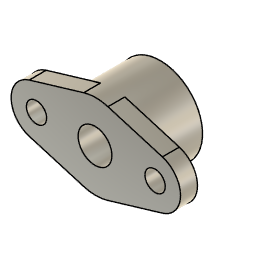
ex 4.1 v0 (Autodesk Fusion 360 design; units mm, degrees)
Autodesk Fusion 360 part; units mm, degrees
sketch "Sketch1" plane through (0, 0, 0) normal (0, 1, 0) x (1, 0, 0)
  circle A0 centre (0, 0) radius 25
  line L0 (20, 0) -> (35, 0)
  line L1 (7.1429, -23.9579) -> (39.2857, -14.3747)
  line L2 (-2.1697, 26.7343) -> (39.2857, 14.3747)
  arc A1 (39.2857, -14.3747) -> (39.2857, 14.3747) centre (35, 0) ccw
  line L3 (0, -63.6354) -> (0, 71.5668)
  line L4 (-7.1429, -23.9579) -> (-39.2857, -14.3747)
  arc A2 (-39.2857, 14.3747) -> (-39.2857, -14.3747) centre (-35, 0) ccw
  line L5 (2.1697, 26.7343) -> (-39.2857, 14.3747)
  circle A3 centre (0, 0) radius 25
  circle A4 centre (-35, 0) radius 6
  circle A5 centre (35, 0) radius 6
  dimension "d1" = 50
  dimension "d2" = 35
  dimension "d3" = 30
  dimension "d4" = 12
  dimension "d5" = 12
  constraint coincident A0.centre A3.centre
  constraint horizontal L0
  constraint coincident L0.end A1.centre
  constraint tangent A0 L1
  constraint tangent L1 A1
  constraint tangent A0 L2
  constraint tangent L2 A1
  constraint coincident L0.start A1
  constraint coincident A0 L1.start
  constraint vertical L3
  constraint symmetric A0 L3 A3
  constraint symmetric L2.start L3 L5.start
  constraint symmetric L1.end L3 L4.end
  constraint symmetric A1 L3 A2
  constraint symmetric L2.end L3 A2.start
  constraint symmetric L1.start L3 L4.start
  constraint concentric A2 A4
  constraint concentric A1 A5
  measures "d1" diameter of A0
  measures "d2" distance of A0.centre L0.end
  measures "d3" diameter of A1
  measures "d4" diameter of A4
  measures "d5" diameter of A5
extrude "Extrude1" add sketch "Sketch1" along normal blind 10 contours A0 L1 L2 A1 A3 | A0 L4 A2 L5 A3 makes body 1 at (31.6163, 0, 10.1046) makes body 2 at (-31.6163, 0, -10.1046)
sketch "Sketch2" plane through (0, 0, 0) normal (0, 1, 0) x (1, 0, 0)
  circle A0 centre (0, 0) radius 25
  circle A1 centre (0, 0) radius 25
  dimension "d8" = 50
  dimension "d9" = 50
  constraint coincident A0.centre A1.centre
  constraint concentric A0 A1
  measures "d8" diameter of A0
  measures "d9" diameter of A1
extrude "Extrude2" add sketch "Sketch2" along normal blind 38 bodies 1 2
hole "Hole1" at (-0.4637, 38, 0.1546) direction (0, -1, 0) diameter 20 depth 38 tip angle 180 counterbore diameter 30 counterbore depth 6 bodies 1
sketch "Sketch3" plane through (0, 0, 0) normal (0, 0, 1) x (1, 0, 0)
  line L0 (0, 0) -> (0, 26)
  dimension "d17" = 26
  constraint coincident L0.start origin
  constraint vertical L0
  measures "d17" distance of L0.start L0.end
hole "Hole2" at (0, 26, 0) direction (0, 0, -1) diameter 6 depth 25 tip angle 180 bodies 1
